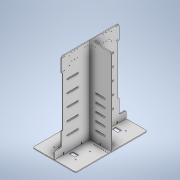
# Autodesk Inventor part: основа
Saved by Autodesk Inventor 2022 (Build 260153000, 153)
## iProperties
Created: 2022-11-18
Part Number: основа
Material: Типовые
Document SubType Name: Modeling
Designer: Ольга
Density: 1 g/cm^3
Appearance: По умолчанию
Author: Ольга
Autodesk Inventor part; units mm, degrees
(part 1 of 2)
sketch "Эскиз1" plane through (0, 0, 0) normal (0, 1, 0) x (-1, 0, 0)
  line L0 (150, 250) -> (-150, 250)
  line L1 (-150, 250) -> (-150, -250)
  line L2 (-150, -250) -> (150, -250)
  line L3 (150, -250) -> (150, 250)
  line L4 (150, 250) -> (-150, -250) construction
  line L5 (-150, 250) -> (150, -250) construction
  line L6 (150, 128.3333) -> (-150, 128.3333) construction
  line L7 (-150, 128.3333) -> (-150, -128.3333) construction
  line L8 (-150, -128.3333) -> (150, -128.3333) construction
  line L9 (150, -128.3333) -> (150, 128.3333) construction
  line L10 (150, 128.3333) -> (-150, -128.3333) construction
  line L11 (-150, 128.3333) -> (150, -128.3333) construction
  line L12 (150, 121.6667) -> (-150, 121.6667) construction
  line L13 (-150, 121.6667) -> (-150, -121.6667) construction
  line L14 (-150, -121.6667) -> (150, -121.6667) construction
  line L15 (150, -121.6667) -> (150, 121.6667) construction
  line L16 (150, 121.6667) -> (-150, -121.6667) construction
  line L17 (-150, 121.6667) -> (150, -121.6667) construction
  line L18 (0, 128.3333) -> (0, 121.6667) construction
  line L19 (0, -121.6667) -> (0, -128.3333) construction
  line L20 (0, 250) -> (0, 125) construction
  line L21 (0, 125) -> (0, 0) construction
  line L22 (0, 0) -> (0, -125) construction
  line L23 (0, -125) -> (0, -250) construction
  circle A0 centre (0, 187.5) radius 2
  circle A1 centre (0, 62.5) radius 2
  circle A2 centre (0, -62.5) radius 2
  circle A3 centre (0, -187.5) radius 2
  line L24 (0, 250) -> (0, 187.5) construction
  line L25 (0, 125) -> (0, 187.5) construction
  line L26 (0, 125) -> (0, 62.5) construction
  line L27 (0, 62.5) -> (0, 0) construction
  line L28 (0, 0) -> (0, -62.5) construction
  line L29 (0, -62.5) -> (0, -125) construction
  line L30 (0, -125) -> (0, -187.5) construction
  line L31 (0, -187.5) -> (0, -250) construction
  line L32 (3, 233.75) -> (-3, 233.75)
  line L33 (-3, 233.75) -> (-3, 203.75)
  line L34 (-3, 203.75) -> (3, 203.75)
  line L35 (3, 203.75) -> (3, 233.75)
  line L36 (3, 233.75) -> (-3, 203.75) construction
  line L37 (-3, 233.75) -> (3, 203.75) construction
  line L38 (3, 171.25) -> (-3, 171.25)
  line L39 (-3, 171.25) -> (-3, 141.25)
  line L40 (-3, 141.25) -> (3, 141.25)
  line L41 (3, 141.25) -> (3, 171.25)
  line L42 (3, 171.25) -> (-3, 141.25) construction
  line L43 (-3, 171.25) -> (3, 141.25) construction
  line L44 (3, 108.75) -> (-3, 108.75)
  line L45 (-3, 108.75) -> (-3, 78.75)
  line L46 (-3, 78.75) -> (3, 78.75)
  line L47 (3, 78.75) -> (3, 108.75)
  line L48 (3, 108.75) -> (-3, 78.75) construction
  line L49 (-3, 108.75) -> (3, 78.75) construction
  line L50 (3, 46.25) -> (-3, 46.25)
  line L51 (-3, 46.25) -> (-3, 16.25)
  line L52 (-3, 16.25) -> (3, 16.25)
  line L53 (3, 16.25) -> (3, 46.25)
  line L54 (3, 46.25) -> (-3, 16.25) construction
  line L55 (-3, 46.25) -> (3, 16.25) construction
  line L56 (3, -16.25) -> (-3, -16.25)
  line L57 (-3, -16.25) -> (-3, -46.25)
  line L58 (-3, -46.25) -> (3, -46.25)
  line L59 (3, -46.25) -> (3, -16.25)
  line L60 (3, -16.25) -> (-3, -46.25) construction
  line L61 (-3, -16.25) -> (3, -46.25) construction
  line L62 (3, -78.75) -> (-3, -78.75)
  line L63 (-3, -78.75) -> (-3, -108.75)
  line L64 (-3, -108.75) -> (3, -108.75)
  line L65 (3, -108.75) -> (3, -78.75)
  line L66 (3, -78.75) -> (-3, -108.75) construction
  line L67 (-3, -78.75) -> (3, -108.75) construction
  line L68 (3, -141.25) -> (-3, -141.25)
  line L69 (-3, -141.25) -> (-3, -171.25)
  line L70 (-3, -171.25) -> (3, -171.25)
  line L71 (3, -171.25) -> (3, -141.25)
  line L72 (3, -141.25) -> (-3, -171.25) construction
  line L73 (-3, -141.25) -> (3, -171.25) construction
  line L74 (3, -203.75) -> (-3, -203.75)
  line L75 (-3, -203.75) -> (-3, -233.75)
  line L76 (-3, -233.75) -> (3, -233.75)
  line L77 (3, -233.75) -> (3, -203.75)
  line L78 (3, -203.75) -> (-3, -233.75) construction
  line L79 (-3, -203.75) -> (3, -233.75) construction
  line L80 (0, 0) -> (-150, 0) construction
  line L81 (-75, 0) -> (0, 0) construction
  line L82 (-75, 0) -> (-150, 0) construction
  line L83 (0, 0) -> (150, 0) construction
  line L84 (75, 0) -> (150, 0) construction
  line L85 (75, 0) -> (0, 0) construction
  line L86 (-97.5, 3) -> (-127.5, 3)
  line L87 (-127.5, 3) -> (-127.5, -3)
  line L88 (-127.5, -3) -> (-97.5, -3)
  line L89 (-97.5, -3) -> (-97.5, 3)
  line L90 (-97.5, 3) -> (-127.5, -3) construction
  line L91 (-127.5, 3) -> (-97.5, -3) construction
  line L92 (-22.5, 3) -> (-52.5, 3)
  line L93 (-52.5, 3) -> (-52.5, -3)
  line L94 (-52.5, -3) -> (-22.5, -3)
  line L95 (-22.5, -3) -> (-22.5, 3)
  line L96 (-22.5, 3) -> (-52.5, -3) construction
  line L97 (-52.5, 3) -> (-22.5, -3) construction
  line L98 (52.5, 3) -> (22.5, 3)
  line L99 (22.5, 3) -> (22.5, -3)
  line L100 (22.5, -3) -> (52.5, -3)
  line L101 (52.5, -3) -> (52.5, 3)
  line L102 (52.5, 3) -> (22.5, -3) construction
  line L103 (22.5, 3) -> (52.5, -3) construction
  line L104 (127.5, 3) -> (97.5, 3)
  line L105 (97.5, 3) -> (97.5, -3)
  line L106 (97.5, -3) -> (127.5, -3)
  line L107 (127.5, -3) -> (127.5, 3)
  line L108 (127.5, 3) -> (97.5, -3) construction
  line L109 (97.5, 3) -> (127.5, -3) construction
  circle A4 centre (-75, 0) radius 2
  circle A5 centre (75, 0) radius 2
  arc A6 (150, 240) -> (140, 250) centre (140, 240) ccw
  arc A7 (140, -250) -> (150, -240) centre (140, -240) ccw
  arc A8 (-150, -240) -> (-140, -250) centre (-140, -240) ccw
  arc A9 (-140, 250) -> (-150, 240) centre (-140, 240) ccw
  line L110 (-150, 20) -> (-8.6161, 20) construction
  circle A10 centre (-140, 20) radius 2.5
  circle A11 centre (-127.1429, 20) radius 2.5
  circle A12 centre (-114.2857, 20) radius 2.5
  circle A13 centre (-101.4286, 20) radius 2.5
  circle A14 centre (-88.5714, 20) radius 2.5
  circle A15 centre (-75.7143, 20) radius 2.5
  circle A16 centre (-62.8571, 20) radius 2.5
  circle A17 centre (-50, 20) radius 2.5
  circle A18 centre (-140, -20) radius 2.5
  circle A19 centre (-127.1429, -20) radius 2.5
  circle A20 centre (-114.2857, -20) radius 2.5
  circle A21 centre (-101.4286, -20) radius 2.5
  circle A22 centre (-88.5714, -20) radius 2.5
  circle A23 centre (-75.7143, -20) radius 2.5
  circle A24 centre (-62.8571, -20) radius 2.5
  circle A25 centre (-50, -20) radius 2.5
  line L111 (0, 125) -> (150, 125) construction
  line L112 (0, -125) -> (150, -125) construction
  circle A26 centre (35, 125) radius 2.5
  circle A27 centre (35, -125) radius 2.5
  point P0 (0, 218.75)
  point P1 (0, 156.25)
  point P2 (0, 93.75)
  point P3 (0, 31.25)
  point P4 (0, -31.25)
  point P5 (0, -93.75)
  point P6 (0, -156.25)
  point P7 (0, -218.75)
  point P8 (0, 156.25)
  point P9 (0, 93.75)
  point P10 (0, 31.25)
  point P11 (0, -31.25)
  point P12 (0, -93.75)
  point P13 (0, -156.25)
  point P14 (0, -218.75)
  point P15 (-112.5, 0)
  point P16 (-37.5, 0)
  point P17 (37.5, 0)
  point P18 (112.5, 0)
  point P19 (-37.5, 0)
  point P20 (37.5, 0)
  point P21 (112.5, 0)
  dimension "d0" = 300
  dimension "d1" = 500
  dimension "d2" = 256.6667
  dimension "d3" = 243.3333
  dimension "d6" = 4
  dimension "d7" = 4
  dimension "d8" = 4
  dimension "d9" = 4
  dimension "d10" = 6
  dimension "d11" = 30
  dimension "d17" = 6
  dimension "d18" = 30
  dimension "d19" = 6
  dimension "d20" = 30
  dimension "d21" = 6
  dimension "d22" = 30
  dimension "d23" = 6
  dimension "d24" = 30
  dimension "d25" = 6
  dimension "d26" = 30
  dimension "d27" = 6
  dimension "d28" = 30
  dimension "d29" = 6
  dimension "d30" = 30
  dimension "d33" = 30
  dimension "d34" = 6
  dimension "d35" = 30
  dimension "d36" = 6
  dimension "d37" = 30
  dimension "d38" = 6
  dimension "d39" = 30
  dimension "d40" = 6
  dimension "d41" = 4
  dimension "d62" = 4
  dimension "d122" = 10
  dimension "d125" = 280
  dimension "d128" = 480
  dimension "d198" = 20
  dimension "d199" = 5
  dimension "d209" = 10
  dimension "d212" = 12.8571
  dimension "d235" = 16.25
  dimension "d236" = 5
  dimension "d237" = 35
  constraints: 226 end point, 58 midpoint, 30 parallel, 28 centre point, 19 horizontal, 17 perpendicular, 15 point on line, 12 collinear, 9 symmetric about line, 8 point on circle, 7 tangent, 5 coincident, 2 vertical, 26 other
  measures "d0" distance of L2.end L1.end
  measures "d1" distance of L1.end L0.end
  measures "d2" distance of L7.end L6.end
  measures "d3" distance of L13.end L12.end
  measures "d6" diameter of A0
  measures "d7" diameter of A1
  measures "d8" diameter of A2
  measures "d9" diameter of A3
  measures "d10" distance of L34.end L33.end
  measures "d11" distance of L33.end L32.end
  measures "d17" distance of L40.end L40.start
  measures "d18" distance of L40.start L39.start
  measures "d19" distance of L46.end L46.start
  measures "d20" distance of L46.start L45.start
  measures "d21" distance of L52.end L52.start
  measures "d22" distance of L52.start L51.start
  measures "d23" distance of L58.end L58.start
  measures "d24" distance of L58.start L57.start
  measures "d25" distance of L64.end L64.start
  measures "d26" distance of L64.start L63.start
  measures "d27" distance of L70.end L70.start
  measures "d28" distance of L70.start L69.start
  measures "d29" distance of L76.end L76.start
  measures "d30" distance of L76.start L75.start
  measures "d33" distance of L88.end L87.end
  measures "d34" distance of L87.end L86.end
  measures "d35" distance of L94.end L94.start
  measures "d36" distance of L94.start L92.end
  measures "d37" distance of L100.end L100.start
  measures "d38" distance of L100.start L98.end
  measures "d39" distance of L106.end L106.start
  measures "d40" distance of L106.start L104.end
  measures "d41" diameter of A4
  measures "d62" diameter of A5
  measures "d122" radius of A6
  measures "d125" distance of A6.centre point (-140, 240)
  measures "d128" distance of A6.centre point (140, -240)
  measures "d198" distance of L110.start L80.end
  measures "d199" diameter of A10
  measures "d209" distance of L110.start A10.centre
  measures "d212" distance of A10.centre A11.centre
  measures "d235" distance from line of L21.end L52
  measures "d236" diameter of A26
  measures "d237" distance of A26.centre L20.end
extrude "Выдавливание1" add sketch "Эскиз1" along normal blind 6 contours A6 L3 A7 L2 A8 L1 A9 L0
ref_plane "РабПлоскость1" through (0, 0, 108.75) normal (1, 0, 0) x (0, 0, -1)
sketch "Эскиз2" plane through (0, 0, 108.75) normal (1, 0, 0) x (0, 0, -1)
  line L0 (294.25, 6) -> (298.25, 6) projected
  line L1 (-80.75, 6) -> (-76.75, 6) construction
  line L2 (348.75, 6) -> (-131.25, 6) construction
  line L3 (44.25, 6) -> (48.25, 6) construction
  line L4 (169.25, 6) -> (173.25, 6) construction
  line L5 (171.25, 6) -> (171.25, 32.7871) construction
  line L6 (46.25, 6) -> (46.25, 27.5686) construction
  line L7 (-80.75, 6) -> (-76.75, 6) construction
  line L8 (-78.75, 6) -> (-78.75, 26.6355) construction
  line L9 (294.25, 6) -> (298.25, 6)
  line L10 (298.25, 6) -> (298.25, 21)
  line L11 (298.25, 21) -> (294.25, 21)
  line L12 (294.25, 21) -> (294.25, 6)
  line L13 (296.25, 21) -> (296.25, 6)
  line L14 (292.83, 12.1) -> (299.67, 12.1)
  line L15 (299.67, 12.1) -> (299.67, 9)
  line L16 (299.67, 9) -> (292.83, 9)
  line L17 (292.83, 9) -> (292.83, 12.1)
  line L18 (292.83, 12.1) -> (299.67, 9) construction
  line L19 (299.67, 12.1) -> (292.83, 9) construction
  line L20 (169.25, 6) -> (173.25, 6)
  line L21 (173.25, 6) -> (173.25, 21)
  line L22 (173.25, 21) -> (169.25, 21)
  line L23 (169.25, 21) -> (169.25, 6)
  line L24 (171.25, 21) -> (171.25, 6)
  line L25 (167.83, 12.1) -> (174.67, 12.1)
  line L26 (174.67, 12.1) -> (174.67, 9)
  line L27 (174.67, 9) -> (167.83, 9)
  line L28 (167.83, 9) -> (167.83, 12.1)
  line L29 (167.83, 12.1) -> (174.67, 9) construction
  line L30 (174.67, 12.1) -> (167.83, 9) construction
  line L31 (44.25, 6) -> (48.25, 6)
  line L32 (48.25, 6) -> (48.25, 21)
  line L33 (48.25, 21) -> (44.25, 21)
  line L34 (44.25, 21) -> (44.25, 6)
  line L35 (46.25, 21) -> (46.25, 6)
  line L36 (42.83, 12.1) -> (49.67, 12.1)
  line L37 (49.67, 12.1) -> (49.67, 9)
  line L38 (49.67, 9) -> (42.83, 9)
  line L39 (42.83, 9) -> (42.83, 12.1)
  line L40 (42.83, 12.1) -> (49.67, 9) construction
  line L41 (49.67, 12.1) -> (42.83, 9) construction
  line L42 (-80.75, 6) -> (-76.75, 6)
  line L43 (-76.75, 6) -> (-76.75, 21)
  line L44 (-76.75, 21) -> (-80.75, 21)
  line L45 (-80.75, 21) -> (-80.75, 6)
  line L46 (-78.75, 21) -> (-78.75, 6)
  line L47 (-82.15, 12.1) -> (-75.35, 12.1)
  line L48 (-75.35, 12.1) -> (-75.35, 9)
  line L49 (-75.35, 9) -> (-82.15, 9)
  line L50 (-82.15, 9) -> (-82.15, 12.1)
  line L51 (-82.15, 12.1) -> (-75.35, 9) construction
  line L52 (-75.35, 12.1) -> (-82.15, 9) construction
  line L53 (-141.25, 6) -> (358.75, 6)
  line L54 (358.75, 6) -> (358.75, 596)
  line L55 (348.75, 606) -> (-131.25, 606)
  line L56 (-141.25, 596) -> (-141.25, 6)
  line L57 (-131.25, 6) -> (348.75, 6) projected
  line L58 (108.75, 606) -> (108.75, 6) construction
  line L59 (-141.25, 6) -> (358.75, 6)
  line L60 (108.75, 606) -> (111.75, 606)
  line L61 (111.75, 606) -> (111.75, 306)
  line L62 (111.75, 306) -> (105.75, 306)
  line L63 (105.75, 306) -> (105.75, 606)
  arc A0 (-131.25, 606) -> (-141.25, 596) centre (-131.25, 596) ccw
  arc A1 (358.75, 596) -> (348.75, 606) centre (348.75, 596) ccw
  point P0 (296.25, 10.55)
  point P1 (171.25, 11.55)
  point P2 (46.25, 11.55)
  point P3 (-78.75, 11.55)
  point P4 (171.25, 10.55)
  point P5 (46.25, 10.55)
  point P6 (-78.75, 10.55)
  point P7 (358.75, 606)
  point P8 (-141.25, 606)
  point P9 (44.25, 12.1)
  point P10 (48.25, 12.1)
  point P11 (48.25, 9)
  point P12 (48.25, 6)
  point P13 (169.25, 9)
  point P14 (169.25, 12.1)
  point P15 (173.25, 12.1)
  point P16 (173.25, 9)
  point P17 (173.25, 6)
  point P18 (294.25, 9)
  point P19 (294.25, 12.1)
  point P20 (298.25, 12.1)
  point P21 (298.25, 9)
  point P22 (-80.75, 9)
  point P23 (-80.75, 12.1)
  point P24 (-76.75, 12.1)
  point P25 (-76.75, 9)
  point P26 (44.25, 6)
  point P27 (44.25, 9)
  point P28 (235.75, 6)
  point P29 (-14.25, 6)
  dimension "d64" = 15
  dimension "d65" = 6.84
  dimension "d66" = 3.1
  dimension "d67" = 3
  dimension "d71" = 15
  dimension "d72" = 6.84
  dimension "d73" = 3.1
  dimension "d74" = 15
  dimension "d75" = 6.84
  dimension "d76" = 3.1
  dimension "d80" = 15
  dimension "d81" = 6.8
  dimension "d82" = 3.1
  dimension "d83" = 600
  dimension "d143" = 3
  dimension "d144" = 300
  dimension "d145" = 6
  dimension "d146" = 300
  dimension "d147" = 3
  dimension "d148" = 3
  dimension "d149" = 3
  dimension "d150" = 10
  dimension "d151" = 10
  constraints: 116 end point, 20 midpoint, 18 parallel, 13 point on line, 11 horizontal, 9 perpendicular, 4 point on circle, 4 tangent, 4 vertical, 2 centre point, 1 collinear, 3 other
  measures "d64" distance of L0.end L10.end
  measures "d65" distance of L15.end L16.end
  measures "d66" distance of L14.end L15.end
  measures "d71" distance of L4.end L21.end
  measures "d72" distance of L26.end L28.start
  measures "d73" distance of L26.start L26.end
  measures "d74" distance of L3.end L32.end
  measures "d75" distance of L37.end L39.start
  measures "d76" distance of L37.start L37.end
  measures "d80" distance of L1.end L43.end
  measures "d81" distance of L48.end L50.start
  measures "d82" distance of L48.start L48.end
  measures "d83" distance of L53.end point (358.75, 606)
  measures "d143" distance of L58.start L60.end
  measures "d144" distance of L60.end L61.end
  measures "d145" distance of L61.end L62.end
  measures "d146" distance of L62.end L63.end
  measures "d147" distance from line of L1.end L49
  measures "d150" radius of A0
  measures "d151" radius of A1
extrude "Выдавливание2" add sketch "Эскиз2" along normal mid plane 6 separate body contours L53 L21 L27 L26 L25 L22 L23 L28 L32 L38 L37 L36 L33 L34 L39 L43 L49 L48 L47 L44 L45 L50 L56 A0 L55 L63 L62 L61 A1 L54 L10 L16 L15 L14 L11 L12 L17
ref_plane "РабПлоскость2" through (22.5, 0, 0) normal (0, 0, 1) x (1, 0, 0)
sketch "Эскиз4" plane through (22.5, 0, 0) normal (0, 0, 1) x (1, 0, 0)
  line L0 (117.5, 6) -> (-162.5, 6) construction
  line L1 (-172.5, 6) -> (127.5, 6)
  line L2 (127.5, 6) -> (127.5, 596)
  line L3 (117.5, 606) -> (-162.5, 606)
  line L4 (-172.5, 596) -> (-172.5, 6)
  line L5 (-19.5, 6) -> (-19.5, 306)
  line L6 (-19.5, 306) -> (-25.5, 306)
  line L7 (-25.5, 306) -> (-25.5, 6)
  arc A0 (-162.5, 606) -> (-172.5, 596) centre (-162.5, 596) ccw
  arc A1 (127.5, 596) -> (117.5, 606) centre (117.5, 596) ccw
  line L8 (-162.5, 6) -> (117.5, 6) projected
  line L9 (-22.5, 606) -> (-22.5, 6) construction
  line L10 (-99.5, 6) -> (-95.5, 6) projected
  line L11 (-99.5, 6) -> (-99.5, 19)
  line L12 (-99.5, 6) -> (-99.5, 0) projected
  line L13 (-99.5, 19) -> (-95.5, 19)
  line L14 (-95.5, 19) -> (-95.5, 6)
  line L15 (-100.9, 12.1) -> (-94.1, 12.1)
  line L16 (-94.1, 12.1) -> (-94.1, 9)
  line L17 (-94.1, 9) -> (-100.9, 9)
  line L18 (-100.9, 9) -> (-100.9, 12.1)
  line L19 (-100.9, 12.1) -> (-94.1, 9) construction
  line L20 (-94.1, 12.1) -> (-100.9, 9) construction
  line L21 (-97.5, 19) -> (-97.5, 6) construction
  line L22 (50.5, 6) -> (50.5, 19)
  line L23 (50.5, 19) -> (54.5, 19)
  line L24 (54.5, 19) -> (54.5, 6)
  line L25 (49.1, 12.1) -> (55.9, 12.1)
  line L26 (55.9, 12.1) -> (55.9, 9)
  line L27 (55.9, 9) -> (49.1, 9)
  line L28 (49.1, 9) -> (49.1, 12.1)
  line L29 (49.1, 12.1) -> (55.9, 9) construction
  line L30 (55.9, 12.1) -> (49.1, 9) construction
  line L31 (52.5, 19) -> (52.5, 6) construction
  line L32 (50.5, 6) -> (54.5, 6) construction
  line L33 (50.5, 6) -> (54.5, 6) construction
  line L34 (50.5, 6) -> (54.5, 6)
  line L35 (-172.5, 0) -> (-172.5, 6) projected
  line L36 (127.5, 0) -> (127.5, 6) projected
  line L37 (-25.5, 606) -> (-19.5, 606) projected
  line L38 (-25.5, 606) -> (-19.5, 606) projected
  line L39 (-19.5, 596) -> (-19.5, 606) projected
  line L40 (-25.5, 606) -> (-19.5, 606)
  point P0 (127.5, 606)
  point P1 (-172.5, 606)
  point P2 (-22.5, 306)
  point P3 (-97.5, 10.55)
  point P4 (-97.5, 10.55)
  point P5 (52.5, 10.55)
  point P6 (52.5, 10.55)
  point P7 (-99.5, 9)
  point P8 (-99.5, 12.1)
  point P9 (-95.5, 12.1)
  point P10 (-95.5, 9)
  point P11 (50.5, 9)
  point P12 (50.5, 12.1)
  point P13 (54.5, 12.1)
  point P14 (54.5, 9)
  dimension "d120" = 10
  dimension "d121" = 10
  dimension "d131" = 13
  dimension "d132" = 6.8
  dimension "d133" = 3.1
  dimension "d134" = 3
  dimension "d135" = 13
  dimension "d136" = 6.8
  dimension "d137" = 3.1
  dimension "d138" = 3
  constraints: 62 end point, 13 midpoint, 7 parallel, 7 point on line, 5 perpendicular, 4 collinear, 4 point on circle, 4 tangent, 3 horizontal, 3 vertical, 2 centre point, 1 other
  measures "d120" radius of A0
  measures "d121" radius of A1
  measures "d131" distance of L10.start L11.end
  measures "d132" distance of L16.end L17.end
  measures "d133" distance of L15.end L16.end
  measures "d134" distance from line of L10.end L17
  measures "d135" distance of L22.start L22.end
  measures "d136" distance of L26.end L30.end
  measures "d137" distance of L26.start L26.end
  measures "d138" distance from line of L24.end L27
extrude "Выдавливание3" add sketch "Эскиз4" along normal mid plane 6 separate body contours L4 A0 L3 A1 L2 L1 L24 L27 L26 L25 L23 L22 L28 L5 L6 L7 L14 L17 L16 L15 L13 L11 L18
sketch "Эскиз5" plane through (-150, 6, 3) normal (0, -1, 0) x (1, 0, 0)
  line L0 (300, 237) -> (300, -243) projected
  line L1 (10, 247) -> (290, 247) projected
  line L2 (0, -243) -> (0, 237) projected
  line L3 (290, -253) -> (10, -253) projected
  circle A0 centre (75, -3) radius 2 projected
  circle A1 centre (225, -3) radius 2 projected
  circle A2 centre (150, -190.5) radius 2 projected
  circle A3 centre (150, -65.5) radius 2 projected
  circle A4 centre (150, 59.5) radius 2 projected
  circle A5 centre (150, 184.5) radius 2 projected
  line L4 (22.5, 0) -> (22.5, -6) projected
  line L5 (52.5, 0) -> (22.5, 0) projected
  line L6 (52.5, -6) -> (52.5, 0) projected
  line L7 (22.5, -6) -> (52.5, -6) projected
  line L8 (97.5, 0) -> (97.5, -6) projected
  line L9 (127.5, 0) -> (97.5, 0) projected
  line L10 (127.5, -6) -> (127.5, 0) projected
  line L11 (97.5, -6) -> (127.5, -6) projected
  line L12 (172.5, 0) -> (172.5, -6) projected
  line L13 (202.5, 0) -> (172.5, 0) projected
  line L14 (202.5, -6) -> (202.5, 0) projected
  line L15 (172.5, -6) -> (202.5, -6) projected
  line L16 (247.5, 0) -> (247.5, -6) projected
  line L17 (277.5, 0) -> (247.5, 0) projected
  line L18 (277.5, -6) -> (277.5, 0) projected
  line L19 (247.5, -6) -> (277.5, -6) projected
  line L20 (153, -236.75) -> (153, -206.75) projected
  line L21 (147, -236.75) -> (153, -236.75) projected
  line L22 (147, -206.75) -> (147, -236.75) projected
  line L23 (153, -206.75) -> (147, -206.75) projected
  line L24 (153, -174.25) -> (153, -144.25) projected
  line L25 (147, -174.25) -> (153, -174.25) projected
  line L26 (147, -144.25) -> (147, -174.25) projected
  line L27 (153, -144.25) -> (147, -144.25) projected
  line L28 (153, -111.75) -> (153, -81.75) projected
  line L29 (147, -111.75) -> (153, -111.75) projected
  line L30 (147, -81.75) -> (147, -111.75) projected
  line L31 (153, -81.75) -> (147, -81.75) projected
  line L32 (153, -49.25) -> (153, -19.25) projected
  line L33 (147, -49.25) -> (153, -49.25) projected
  line L34 (147, -19.25) -> (147, -49.25) projected
  line L35 (153, -19.25) -> (147, -19.25) projected
  line L36 (153, 13.25) -> (153, 43.25) projected
  line L37 (147, 13.25) -> (153, 13.25) projected
  line L38 (147, 43.25) -> (147, 13.25) projected
  line L39 (153, 43.25) -> (147, 43.25) projected
  line L40 (153, 75.75) -> (153, 105.75) projected
  line L41 (147, 75.75) -> (153, 75.75) projected
  line L42 (147, 105.75) -> (147, 75.75) projected
  line L43 (153, 105.75) -> (147, 105.75) projected
  line L44 (153, 138.25) -> (153, 168.25) projected
  line L45 (147, 138.25) -> (153, 138.25) projected
  line L46 (147, 168.25) -> (147, 138.25) projected
  line L47 (153, 168.25) -> (147, 168.25) projected
  line L48 (147, 230.75) -> (147, 200.75) projected
  line L49 (153, 230.75) -> (147, 230.75) projected
  line L50 (153, 200.75) -> (153, 230.75) projected
  line L51 (147, 200.75) -> (153, 200.75) projected
  line L52 (153, -236.75) -> (147, -236.75)
  line L53 (147, -236.75) -> (147, -206.75)
  line L54 (147, -206.75) -> (153, -206.75)
  line L55 (153, -206.75) -> (153, -236.75)
  line L56 (147, -144.25) -> (153, -144.25)
  line L57 (147, -174.25) -> (147, -144.25)
  line L58 (153, -174.25) -> (147, -174.25)
  line L59 (153, -144.25) -> (153, -174.25)
  line L60 (147, -81.75) -> (153, -81.75)
  line L61 (147, -111.75) -> (147, -81.75)
  line L62 (153, -111.75) -> (147, -111.75)
  line L63 (153, -81.75) -> (153, -111.75)
  line L64 (147, -19.25) -> (153, -19.25)
  line L65 (147, -49.25) -> (147, -19.25)
  line L66 (153, -49.25) -> (147, -49.25)
  line L67 (153, -19.25) -> (153, -49.25)
  line L68 (147, 43.25) -> (153, 43.25)
  line L69 (147, 13.25) -> (147, 43.25)
  line L70 (153, 13.25) -> (147, 13.25)
  line L71 (153, 43.25) -> (153, 13.25)
  line L72 (147, 105.75) -> (153, 105.75)
  line L73 (147, 75.75) -> (147, 105.75)
  line L74 (153, 75.75) -> (147, 75.75)
  line L75 (153, 105.75) -> (153, 75.75)
  line L76 (147, 168.25) -> (153, 168.25)
  line L77 (147, 138.25) -> (147, 168.25)
  line L78 (153, 138.25) -> (147, 138.25)
  line L79 (153, 168.25) -> (153, 138.25)
  line L80 (147, 230.75) -> (153, 230.75)
  line L81 (147, 200.75) -> (147, 230.75)
  line L82 (153, 200.75) -> (147, 200.75)
  line L83 (153, 230.75) -> (153, 200.75)
  line L84 (277.5, 0) -> (247.5, 0)
  line L85 (247.5, 0) -> (247.5, -6)
  line L86 (247.5, -6) -> (277.5, -6)
  line L87 (277.5, -6) -> (277.5, 0)
  line L88 (172.5, 0) -> (172.5, -6)
  line L89 (202.5, 0) -> (172.5, 0)
  line L90 (172.5, -6) -> (202.5, -6)
  line L91 (202.5, -6) -> (202.5, 0)
  line L92 (97.5, 0) -> (97.5, -6)
  line L93 (127.5, 0) -> (97.5, 0)
  line L94 (97.5, -6) -> (127.5, -6)
  line L95 (127.5, -6) -> (127.5, 0)
  line L96 (22.5, 0) -> (22.5, -6)
  line L97 (52.5, 0) -> (22.5, 0)
  line L98 (22.5, -6) -> (52.5, -6)
  line L99 (52.5, -6) -> (52.5, 0)
  arc A6 (300, 237) -> (290, 247) centre (290, 237) ccw projected
  arc A7 (10, 247) -> (0, 237) centre (10, 237) ccw projected
  arc A8 (0, -243) -> (10, -253) centre (10, -243) ccw projected
  arc A9 (290, -253) -> (300, -243) centre (290, -243) ccw projected
  point P0 (150, -3)
  dimension "d104" = 62.5
  dimension "d111" = 75
  constraints: 96 end point, 4 parallel, 3 horizontal, 2 coincident, 2 perpendicular, 1 vertical, 80 other
  measures "d104" distance of L22.start L56.start
  measures "d111" distance of L84.end L88.start
extrude "Выдавливание4" add sketch "Эскиз5" along normal up to surface (6 mm away) contours L21 L22 L23 L20 | L25 L26 L27 L24 | L29 L30 L31 L28 | L33 L34 L35 L32 | L37 L38 L39 L36 | L41 L42 L43 L40 | L45 L46 L47 L44 | L49 L50 L51 L48 bodies 2
extrude "Выдавливание5" add sketch "Эскиз5" along normal up to surface (6 mm away) contours L5 L6 L7 L4 | L9 L10 L11 L8 | L13 L14 L15 L12 | L17 L18 L19 L16 bodies 3
sketch "Эскиз6" plane through (22.5, 0, 3) normal (0, 0, 1) x (1, 0, 0)
  line L0 (52.5, 6) -> (52.5, 606) construction
  line L1 (50.5, 6) -> (54.5, 6) construction
  line L2 (50.5, 0) -> (54.5, 0) construction
  line L3 (22.5, 81) -> (82.5, 81) construction
  line L4 (22.5, 76) -> (82.5, 76)
  line L5 (82.5, 86) -> (22.5, 86)
  arc A0 (22.5, 86) -> (22.5, 76) centre (22.5, 81) ccw
  arc A1 (82.5, 76) -> (82.5, 86) centre (82.5, 81) ccw
  line L6 (22.5, 137.25) -> (82.5, 137.25) construction
  line L7 (22.5, 132.25) -> (82.5, 132.25)
  line L8 (82.5, 142.25) -> (22.5, 142.25)
  arc A2 (22.5, 142.25) -> (22.5, 132.25) centre (22.5, 137.25) ccw
  arc A3 (82.5, 132.25) -> (82.5, 142.25) centre (82.5, 137.25) ccw
  line L9 (22.5, 193.5) -> (82.5, 193.5) construction
  line L10 (22.5, 188.5) -> (82.5, 188.5)
  line L11 (82.5, 198.5) -> (22.5, 198.5)
  arc A4 (22.5, 198.5) -> (22.5, 188.5) centre (22.5, 193.5) ccw
  arc A5 (82.5, 188.5) -> (82.5, 198.5) centre (82.5, 193.5) ccw
  line L12 (22.5, 249.75) -> (82.5, 249.75) construction
  line L13 (22.5, 244.75) -> (82.5, 244.75)
  line L14 (82.5, 254.75) -> (22.5, 254.75)
  arc A6 (22.5, 254.75) -> (22.5, 244.75) centre (22.5, 249.75) ccw
  arc A7 (82.5, 244.75) -> (82.5, 254.75) centre (82.5, 249.75) ccw
  line L15 (22.5, 306) -> (82.5, 306) construction
  line L16 (22.5, 301) -> (82.5, 301)
  line L17 (82.5, 311) -> (22.5, 311)
  arc A8 (22.5, 311) -> (22.5, 301) centre (22.5, 306) ccw
  arc A9 (82.5, 301) -> (82.5, 311) centre (82.5, 306) ccw
  line L18 (-162.5, 606) -> (117.5, 606) projected
  point P0 (-22.5, 0)
  point P1 (52.5, 81)
  point P2 (52.5, 137.25)
  point P3 (52.5, 193.5)
  point P4 (52.5, 249.75)
  point P5 (52.5, 306)
  point P6 (52.5, 306)
  dimension "d155" = 70
  dimension "d157" = 60
  dimension "d161" = 56.25
  dimension "d170" = 10
  constraints: 42 end point, 20 point on circle, 10 centre point, 4 midpoint, 4 tangent, 2 point on line, 2 vertical, 1 parallel, 1 perpendicular, 48 other
  measures "d155" distance from line of L0.start L4
  measures "d157" distance of L5.start L5.end
  measures "d161" distance of L4.start L7.start
  measures "d170" distance between parallel lines of L5 L4
extrude "Выдавливание6" cut sketch "Эскиз6" against normal blind 6 bodies 3
sketch "Эскиз7" plane through (3, 0, 108.75) normal (1, 0, 0) x (0, 0, -1)
  line L0 (44.25, 6) -> (48.25, 6) construction
  line L1 (44.25, 0) -> (48.25, 0) construction
  line L2 (-80.75, 6) -> (-76.75, 6) construction
  line L3 (-80.75, 0) -> (-76.75, 0) construction
  line L4 (-76.75, 6) -> (44.25, 6) construction
  line L5 (-16.25, 6) -> (-16.25, 606) construction
  line L6 (-131.25, 606) -> (105.75, 606) construction
  line L7 (-51.25, 451) -> (18.75, 451) construction
  line L8 (-51.25, 446) -> (18.75, 446)
  line L9 (18.75, 456) -> (-51.25, 456)
  arc A0 (-51.25, 456) -> (-51.25, 446) centre (-51.25, 451) ccw
  arc A1 (18.75, 446) -> (18.75, 456) centre (18.75, 451) ccw
  line L10 (-51.25, 361) -> (18.75, 361)
  line L11 (-51.25, 366) -> (18.75, 366) construction
  arc A2 (-51.25, 371) -> (-51.25, 361) centre (-51.25, 366) ccw
  arc A3 (18.75, 361) -> (18.75, 371) centre (18.75, 366) ccw
  line L12 (18.75, 371) -> (-51.25, 371)
  line L13 (-51.25, 276) -> (18.75, 276)
  line L14 (-51.25, 281) -> (18.75, 281) construction
  arc A4 (-51.25, 286) -> (-51.25, 276) centre (-51.25, 281) ccw
  arc A5 (18.75, 276) -> (18.75, 286) centre (18.75, 281) ccw
  line L15 (18.75, 286) -> (-51.25, 286)
  line L16 (-51.25, 191) -> (18.75, 191)
  line L17 (-51.25, 196) -> (18.75, 196) construction
  arc A6 (-51.25, 201) -> (-51.25, 191) centre (-51.25, 196) ccw
  arc A7 (18.75, 191) -> (18.75, 201) centre (18.75, 196) ccw
  line L18 (18.75, 201) -> (-51.25, 201)
  line L19 (-51.25, 106) -> (18.75, 106)
  line L20 (-51.25, 111) -> (18.75, 111) construction
  arc A8 (-51.25, 116) -> (-51.25, 106) centre (-51.25, 111) ccw
  arc A9 (18.75, 106) -> (18.75, 116) centre (18.75, 111) ccw
  line L21 (18.75, 116) -> (-51.25, 116)
  line L22 (198.75, 446) -> (268.75, 446)
  line L23 (198.75, 451) -> (268.75, 451) construction
  arc A10 (198.75, 456) -> (198.75, 446) centre (198.75, 451) ccw
  arc A11 (268.75, 446) -> (268.75, 456) centre (268.75, 451) ccw
  line L24 (268.75, 456) -> (198.75, 456)
  line L25 (198.75, 361) -> (268.75, 361)
  line L26 (198.75, 366) -> (268.75, 366) construction
  arc A12 (198.75, 371) -> (198.75, 361) centre (198.75, 366) ccw
  arc A13 (268.75, 361) -> (268.75, 371) centre (268.75, 366) ccw
  line L27 (268.75, 371) -> (198.75, 371)
  line L28 (198.75, 276) -> (268.75, 276)
  line L29 (198.75, 281) -> (268.75, 281) construction
  arc A14 (198.75, 286) -> (198.75, 276) centre (198.75, 281) ccw
  arc A15 (268.75, 276) -> (268.75, 286) centre (268.75, 281) ccw
  line L30 (268.75, 286) -> (198.75, 286)
  line L31 (198.75, 191) -> (268.75, 191)
  line L32 (198.75, 196) -> (268.75, 196) construction
  arc A16 (198.75, 201) -> (198.75, 191) centre (198.75, 196) ccw
  arc A17 (268.75, 191) -> (268.75, 201) centre (268.75, 196) ccw
  line L33 (268.75, 201) -> (198.75, 201)
  line L34 (198.75, 106) -> (268.75, 106)
  line L35 (198.75, 111) -> (268.75, 111) construction
  arc A18 (198.75, 116) -> (198.75, 106) centre (198.75, 111) ccw
  arc A19 (268.75, 106) -> (268.75, 116) centre (268.75, 111) ccw
  line L36 (268.75, 116) -> (198.75, 116)
  line L37 (233.75, 6) -> (233.75, 658.6053) construction
  line L38 (-76.75, 6) -> (44.25, 6)
  line L39 (348.75, 0) -> (-131.25, 0) projected
  line L40 (173.25, 12.1) -> (173.25, 21) projected
  line L41 (169.25, 6) -> (173.25, 6) projected
  line L42 (294.25, 6) -> (298.25, 6) projected
  line L43 (173.25, 6) -> (294.25, 6)
  point P0 (108.75, 0)
  point P1 (-16.25, 451)
  point P2 (-16.25, 366)
  point P3 (-16.25, 281)
  point P4 (-16.25, 196)
  point P5 (-16.25, 111)
  point P6 (233.75, 451)
  point P7 (233.75, 366)
  point P8 (233.75, 281)
  point P9 (233.75, 196)
  point P10 (233.75, 111)
  point P11 (233.75, 451)
  point P12 (-16.25, 6)
  dimension "d171" = 10
  dimension "d172" = 70
  dimension "d173" = 150
  dimension "d176" = 85
  dimension "d179" = 250
  dimension "d238" = 100
  constraints: 90 end point, 40 point on circle, 20 centre point, 5 midpoint, 4 point on line, 4 tangent, 2 horizontal, 2 parallel, 2 perpendicular, 2 vertical, 108 other
  measures "d171" distance between parallel lines of L8 L9
  measures "d172" distance of L8.start L8.end
  measures "d173" distance between parallel lines of L9 L6
  measures "d176" distance of L8.start L10.start
  measures "d179" distance of L8.start L22.start
  measures "d238" distance between parallel lines of L4 L19
extrude "Выдавливание7" cut sketch "Эскиз7" against normal blind 6 bodies 2
sketch "Эскиз9" plane through (0, 6, 0) normal (0, 1, 0) x (1, 0, 0)
  circle A0 centre (50, -20) radius 2.5 projected
  line L0 (3, -3) -> (3, -240) projected
  line L1 (3, -250) -> (3, -240) projected
  line L2 (-140, -250) -> (140, -250) projected
  arc A1 (140, -250) -> (150, -240) centre (140, -240) ccw projected
  line L3 (150, -240) -> (150, 240) projected
  line L4 (3, -16.25) -> (3, -46.25) construction
  line L5 (3, -22.5) -> (147.0711, -22.5) construction
  line L6 (147.0711, -22.5) -> (147.0711, -247.0711) construction
  line L7 (147.0711, -247.0711) -> (3, -247.0711) construction
  line L8 (3, -247.0711) -> (3, -22.5) construction
  line L9 (137.0711, -32.5) -> (13, -32.5)
  line L10 (13, -32.5) -> (13, -237.0711)
  line L11 (13, -237.0711) -> (137.0711, -237.0711)
  line L12 (137.0711, -237.0711) -> (137.0711, -32.5)
  point P0 (0, 0)
  dimension "d218" = 10
  constraints: 16 end point, 4 parallel, 2 perpendicular, 1 horizontal, 1 point on circle, 1 point on line, 1 tangent, 3 other
  measures "d218" distance between parallel lines of L5 L9
sketch "Эскиз13" plane through (3, 0, 108.75) normal (1, 0, 0) x (0, 0, -1)
  line L0 (198.75, 456) -> (268.75, 456) projected
  arc A0 (268.75, 446) -> (268.75, 456) centre (268.75, 451) ccw projected
  line L1 (268.75, 446) -> (198.75, 446) projected
  arc A1 (198.75, 456) -> (198.75, 446) centre (198.75, 451) ccw projected
  line L2 (198.75, 286) -> (268.75, 286) projected
  arc A2 (268.75, 276) -> (268.75, 286) centre (268.75, 281) ccw projected
  line L3 (268.75, 276) -> (198.75, 276) projected
  arc A3 (198.75, 286) -> (198.75, 276) centre (198.75, 281) ccw projected
  line L4 (-51.25, 456) -> (18.75, 456) projected
  arc A4 (18.75, 446) -> (18.75, 456) centre (18.75, 451) ccw projected
  line L5 (18.75, 446) -> (-51.25, 446) projected
  arc A5 (-51.25, 456) -> (-51.25, 446) centre (-51.25, 451) ccw projected
  line L6 (-51.25, 286) -> (18.75, 286) projected
  arc A6 (18.75, 276) -> (18.75, 286) centre (18.75, 281) ccw projected
  line L7 (18.75, 276) -> (-51.25, 276) projected
  arc A7 (-51.25, 286) -> (-51.25, 276) centre (-51.25, 281) ccw projected
  line L8 (-51.25, 116) -> (18.75, 116) projected
  arc A8 (18.75, 106) -> (18.75, 116) centre (18.75, 111) ccw projected
  line L9 (18.75, 106) -> (-51.25, 106) projected
  arc A9 (-51.25, 116) -> (-51.25, 106) centre (-51.25, 111) ccw projected
  line L10 (-51.25, 201) -> (18.75, 201) projected
  arc A10 (18.75, 191) -> (18.75, 201) centre (18.75, 196) ccw projected
  line L11 (18.75, 191) -> (-51.25, 191) projected
  arc A11 (-51.25, 201) -> (-51.25, 191) centre (-51.25, 196) ccw projected
  line L12 (-51.25, 371) -> (18.75, 371) projected
  arc A12 (18.75, 361) -> (18.75, 371) centre (18.75, 366) ccw projected
  line L13 (18.75, 361) -> (-51.25, 361) projected
  arc A13 (-51.25, 371) -> (-51.25, 361) centre (-51.25, 366) ccw projected
  line L14 (198.75, 201) -> (268.75, 201) projected
  arc A14 (268.75, 191) -> (268.75, 201) centre (268.75, 196) ccw projected
  line L15 (268.75, 191) -> (198.75, 191) projected
  arc A15 (198.75, 201) -> (198.75, 191) centre (198.75, 196) ccw projected
  line L16 (198.75, 371) -> (268.75, 371) projected
  arc A16 (268.75, 361) -> (268.75, 371) centre (268.75, 366) ccw projected
  line L17 (268.75, 361) -> (198.75, 361) projected
  arc A17 (198.75, 371) -> (198.75, 361) centre (198.75, 366) ccw projected
  line L18 (198.75, 116) -> (268.75, 116) projected
  arc A18 (268.75, 106) -> (268.75, 116) centre (268.75, 111) ccw projected
  line L19 (268.75, 106) -> (198.75, 106) projected
  arc A19 (198.75, 116) -> (198.75, 106) centre (198.75, 111) ccw projected
  line L20 (298.25, 6) -> (312.5, 6) projected
  line L21 (312.5, 6) -> (312.5, 0) projected
  line L22 (342.5, 0) -> (312.5, 0) projected
  line L23 (342.5, 6) -> (342.5, 0) projected
  line L24 (342.5, 6) -> (358.75, 6) projected
  line L25 (358.75, 6) -> (358.75, 596) projected
  arc A20 (358.75, 596) -> (348.75, 606) centre (348.75, 596) ccw projected
  line L26 (348.75, 606) -> (111.75, 606) projected
  line L27 (111.75, 606) -> (111.75, 306) projected
  line L28 (111.75, 306) -> (105.75, 306) projected
  line L29 (105.75, 306) -> (105.75, 606) projected
  line L30 (105.75, 606) -> (-131.25, 606) projected
  arc A21 (-131.25, 606) -> (-141.25, 596) centre (-131.25, 596) ccw projected
  line L31 (-141.25, 596) -> (-141.25, 6) projected
  line L32 (-141.25, 6) -> (-125, 6) projected
  line L33 (-125, 6) -> (-125, 0) projected
  line L34 (-95, 0) -> (-125, 0) projected
  line L35 (-95, 6) -> (-95, 0) projected
  line L36 (-95, 6) -> (-80.75, 6) projected
  line L37 (-76.75, 6) -> (-62.5, 6) projected
  line L38 (-62.5, 6) -> (-62.5, 0) projected
  line L39 (-32.5, 0) -> (-62.5, 0) projected
  line L40 (-32.5, 6) -> (-32.5, 0) projected
  line L41 (280, 6) -> (294.25, 6) projected
  line L42 (173.25, 6) -> (187.5, 6) projected
  line L43 (0, 6) -> (0, 0) projected
  line L44 (30, 0) -> (0, 0) projected
  line L45 (30, 6) -> (30, 0) projected
  line L46 (30, 6) -> (44.25, 6) projected
  line L47 (62.5, 6) -> (62.5, 0) projected
  line L48 (92.5, 0) -> (62.5, 0) projected
  line L49 (92.5, 6) -> (92.5, 0) projected
  line L50 (92.5, 6) -> (125, 6) projected
  line L51 (125, 6) -> (125, 0) projected
  line L52 (155, 0) -> (125, 0) projected
  line L53 (155, 6) -> (155, 0) projected
  line L54 (187.5, 6) -> (187.5, 0) projected
  line L55 (217.5, 0) -> (187.5, 0) projected
  line L56 (217.5, 6) -> (217.5, 0) projected
  line L57 (250, 6) -> (250, 0) projected
  line L58 (280, 0) -> (250, 0) projected
  line L59 (280, 6) -> (280, 0) projected
  line L60 (-141.25, 606) -> (-91.25, 606)
  line L61 (-91.25, 596) -> (-91.25, 66)
  line L62 (-101.25, 56) -> (-131.25, 56)
  line L63 (-141.25, 56) -> (-141.25, 606)
  line L64 (-141.25, 596) -> (-141.25, 6) projected
  line L65 (105.75, 606) -> (-131.25, 606) projected
  line L66 (-141.25, 46) -> (-141.25, 19.6406)
  line L67 (-81.25, 606) -> (-14.25, 606)
  arc A22 (-101.25, 56) -> (-91.25, 66) centre (-101.25, 66) ccw
  arc A23 (-81.25, 606) -> (-91.25, 596) centre (-81.25, 596) ccw
  arc A24 (-131.25, 56) -> (-141.25, 46) centre (-131.25, 46) ccw
  line L68 (111.75, 606) -> (105.75, 606) construction
  line L69 (108.75, 606) -> (108.75, 565.581) construction
  arc A25 (358.75, 596) -> (348.75, 606) centre (348.75, 596) ccw
  line L70 (298.25, 21) -> (294.25, 21)
  line L71 (358.75, 606) -> (308.75, 606)
  line L72 (308.75, 596) -> (308.75, 66)
  line L73 (318.75, 56) -> (348.75, 56)
  line L74 (358.75, 56) -> (358.75, 606)
  line L75 (358.75, 46) -> (358.75, 19.6406)
  line L76 (298.75, 606) -> (231.75, 606)
  arc A26 (308.75, 66) -> (318.75, 56) centre (318.75, 66) ccw
  arc A27 (308.75, 596) -> (298.75, 606) centre (298.75, 596) ccw
  arc A28 (358.75, 46) -> (348.75, 56) centre (348.75, 46) ccw
  line L77 (299.67, 9) -> (298.25, 9) projected
  line L78 (298.25, 9) -> (298.25, 6) projected
  line L79 (-80.75, 6) -> (-80.75, 9) projected
  line L80 (-80.75, 9) -> (-82.15, 9) projected
  line L81 (-82.15, 9) -> (-82.15, 12.1) projected
  line L82 (-82.15, 12.1) -> (-80.75, 12.1) projected
  line L83 (-80.75, 12.1) -> (-80.75, 21) projected
  line L84 (-80.75, 21) -> (-76.75, 21) projected
  line L85 (-76.75, 21) -> (-76.75, 12.1) projected
  line L86 (-76.75, 12.1) -> (-75.35, 12.1) projected
  line L87 (-75.35, 12.1) -> (-75.35, 9) projected
  line L88 (-75.35, 9) -> (-76.75, 9) projected
  line L89 (-76.75, 9) -> (-76.75, 6) projected
  line L90 (-32.5, 6) -> (0, 6) projected
  line L91 (44.25, 6) -> (44.25, 9) projected
  line L92 (44.25, 9) -> (42.83, 9) projected
  line L93 (42.83, 9) -> (42.83, 12.1) projected
  line L94 (42.83, 12.1) -> (44.25, 12.1) projected
  line L95 (44.25, 12.1) -> (44.25, 21) projected
  line L96 (44.25, 21) -> (48.25, 21) projected
  line L97 (48.25, 21) -> (48.25, 12.1) projected
  line L98 (48.25, 12.1) -> (49.67, 12.1) projected
  line L99 (49.67, 12.1) -> (49.67, 9) projected
  line L100 (49.67, 9) -> (48.25, 9) projected
  line L101 (48.25, 9) -> (48.25, 6) projected
  line L102 (48.25, 6) -> (62.5, 6) projected
  line L103 (155, 6) -> (169.25, 6) projected
  line L104 (169.25, 6) -> (169.25, 9) projected
  line L105 (169.25, 9) -> (167.83, 9) projected
  line L106 (167.83, 9) -> (167.83, 12.1) projected
  line L107 (167.83, 12.1) -> (169.25, 12.1) projected
  line L108 (169.25, 12.1) -> (169.25, 21) projected
  line L109 (169.25, 21) -> (173.25, 21) projected
  line L110 (173.25, 21) -> (173.25, 12.1) projected
  line L111 (173.25, 12.1) -> (174.67, 12.1) projected
  line L112 (174.67, 12.1) -> (174.67, 9) projected
  line L113 (174.67, 9) -> (173.25, 9) projected
  line L114 (173.25, 9) -> (173.25, 6) projected
  line L115 (217.5, 6) -> (250, 6) projected
  line L116 (294.25, 6) -> (294.25, 9) projected
  line L117 (294.25, 9) -> (292.83, 9) projected
  line L118 (292.83, 9) -> (292.83, 12.1) projected
  line L119 (292.83, 12.1) -> (294.25, 12.1) projected
  line L120 (294.25, 12.1) -> (294.25, 21) projected
  line L121 (294.25, 21) -> (298.25, 21) projected
  line L122 (298.25, 21) -> (298.25, 12.1) projected
  line L123 (298.25, 12.1) -> (299.67, 12.1) projected
  line L124 (299.67, 12.1) -> (299.67, 9) projected
  point P0 (108.75, 0)
  point P1 (-91.25, 56)
  point P2 (308.75, 56)
  point P3 (-141.25, 46)
  dimension "d223" = 50
  dimension "d224" = 550
  dimension "d225" = 10
  dimension "d226" = 10
  constraints: 28 end point, 16 symmetric about line, 14 point on circle, 14 point on line, 7 centre point, 6 tangent, 2 collinear, 2 parallel, 1 equal radius, 1 horizontal, 1 midpoint, 1 perpendicular, 1 vertical, 4 other
  measures "d223" distance of point (-91.25, 56) L63.start
  measures "d224" distance of L60.end point (-91.25, 56)
  measures "d225" radius of A22
  measures "d226" radius of A23
extrude "Выдавливание11" cut sketch "Эскиз13" against normal up to surface (6 mm away) contours A28 L73 A26 L72 A27 L26 A20 L25 | A23 L61 A22 L62 A24 L31 A21 L30 bodies 2
sketch "Эскиз15" plane through (22.5, 0, 3) normal (0, 0, 1) x (1, 0, 0)
  line L0 (-19.5, 606) -> (-19.5, 306) projected
  line L1 (-19.5, 606) -> (126.0275, 368.404)
  line L2 (127.5, 6) -> (127.5, 596) projected
  line L3 (127.5, 363.1809) -> (127.5, 351.8775)
  line L4 (-19.5, 606) -> (-27.8702, 606)
  line L5 (117.5, 606) -> (-162.5, 606) projected
  arc A0 (127.5, 363.1809) -> (126.0275, 368.404) centre (117.5, 363.1809) ccw
  line L6 (-19.5, 606) -> (127.5, 606)
  line L7 (127.5, 606) -> (127.5, 363.1809)
  line L8 (-25.5, 606) -> (-19.5, 606) construction
  line L9 (-22.5, 606) -> (-22.5, 569.2816) construction
  line L10 (-25.5, 606) -> (-171.0275, 368.404)
  line L11 (-172.5, 6) -> (-172.5, 596)
  line L12 (-162.5, 606) -> (117.5, 606)
  line L13 (-25.5, 606) -> (-172.5, 606)
  line L14 (-172.5, 606) -> (-172.5, 363.1809)
  arc A1 (-171.0275, 368.404) -> (-172.5, 363.1809) centre (-162.5, 363.1809) ccw
  point P0 (-22.5, 0)
  point P1 (127.5, 366)
  dimension "d231" = 230
  dimension "d232" = 10
  constraints: 22 end point, 9 symmetric about line, 6 point on line, 4 point on circle, 2 centre point, 2 tangent, 1 horizontal, 1 midpoint, 1 vertical, 1 other
  measures "d231" distance of L2.end point (127.5, 366)
  measures "d232" radius of A0
extrude "Выдавливание13" cut sketch "Эскиз15" against normal up to surface (6 mm away) contours L10 A1 L11 L14 L13 L5 L4 bodies 3
sketch "Эскиз16" plane through (3, 0, 108.75) normal (1, 0, 0) x (0, 0, -1)
  line L0 (111.75, 606) -> (105.75, 606) projected
  line L1 (105.75, 596) -> (105.75, 606) projected
  line L2 (111.75, 596) -> (105.75, 596) projected
  line L3 (111.75, 606) -> (111.75, 596) projected
  line L4 (-81.25, 606) -> (105.75, 606) construction
  line L5 (105.75, 606) -> (105.75, 583.5) construction
  line L6 (105.75, 6) -> (105.75, 596) construction
  line L7 (105.75, 583.5) -> (91.25, 583.5) construction
  line L8 (91.25, 583.5) -> (71.25, 583.5) construction
  circle A0 centre (71.25, 583.5) radius 2
  circle A1 centre (91.25, 583.5) radius 2
  line L9 (108.75, 606) -> (108.75, 583.5) construction
  circle A2 centre (146.25, 583.5) radius 2
  circle A3 centre (126.25, 583.5) radius 2
  point P0 (108.75, 0)
  dimension "d239" = 22.5
  dimension "d240" = 14.5
  dimension "d241" = 20
  dimension "d242" = 4
  dimension "d243" = 4
  constraints: 8 end point, 4 centre point, 2 coincident, 2 point on line, 2 symmetric about line, 1 midpoint, 1 perpendicular, 1 vertical, 2 other
  measures "d239" distance of L0.end L5.end
  measures "d240" distance of L5.end L7.end
  measures "d241" distance of L7.end L8.end
  measures "d242" diameter of A0
  measures "d243" diameter of A1
sketch "Эскиз17" plane through (22.5, 0, 3) normal (0, 0, 1) x (1, 0, 0)
  line L0 (-19.5, 581.5) -> (-19.5, 585.5) projected
  line L1 (-19.5, 583.5) -> (-5, 583.5) construction
  line L2 (-5, 583.5) -> (15, 583.5) construction
  circle A0 centre (-5, 583.5) radius 2
  circle A1 centre (15, 583.5) radius 2
  point P0 (-22.5, 0)
  dimension "d244" = 14.5
  dimension "d245" = 20
  dimension "d246" = 4
  dimension "d247" = 4
  constraints: 4 end point, 2 centre point, 2 coincident, 2 horizontal, 1 midpoint
  measures "d244" distance of L1.start L1.end
  measures "d245" distance of L1.end L2.end
  measures "d246" diameter of A0
  measures "d247" diameter of A1
extrude "Выдавливание14" cut sketch "Эскиз16" against normal up to surface (6 mm away) contours A0 | A1 | A2 | A3 bodies 2
extrude "Выдавливание15" cut sketch "Эскиз17" against normal up to surface (6 mm away) bodies 3
ref_plane "РабПлоскость3" through (22.5, 0, 0) normal (0, 0, -1) x (-1, 0, 0)
sketch "Эскиз18" plane through (3, 0, 108.75) normal (1, 0, 0) x (0, 0, -1)
  line L0 (-91.25, 66) -> (-91.25, 596) projected
  line L1 (-89.25, 506) -> (-85.75, 506)
  line L2 (-83.75, 504) -> (-83.75, 158)
  line L3 (-85.75, 156) -> (-89.25, 156)
  line L4 (-91.25, 156) -> (-91.25, 506)
  line L5 (105.75, 606) -> (-81.25, 606) projected
  arc A0 (-83.75, 504) -> (-85.75, 506) centre (-85.75, 504) ccw
  line L6 (-91.25, 508) -> (-91.25, 531.208)
  arc A1 (-91.25, 508) -> (-89.25, 506) centre (-89.25, 508) ccw
  arc A2 (-85.75, 156) -> (-83.75, 158) centre (-85.75, 158) ccw
  line L7 (-91.25, 154) -> (-91.25, 127.391)
  arc A3 (-89.25, 156) -> (-91.25, 154) centre (-89.25, 154) ccw
  line L8 (108.75, 727.2) -> (108.75, -121.2) projected
  line L9 (308.75, 66) -> (308.75, 596)
  line L10 (306.75, 506) -> (303.25, 506)
  line L11 (301.25, 504) -> (301.25, 158)
  line L12 (303.25, 156) -> (306.75, 156)
  arc A4 (303.25, 506) -> (301.25, 504) centre (303.25, 504) ccw
  arc A5 (306.75, 506) -> (308.75, 508) centre (306.75, 508) ccw
  arc A6 (301.25, 158) -> (303.25, 156) centre (303.25, 158) ccw
  arc A7 (308.75, 154) -> (306.75, 156) centre (306.75, 154) ccw
  point P0 (108.75, 0)
  point P1 (-83.75, 156)
  point P2 (-83.75, 506)
  point P3 (308.75, 508)
  point P4 (-91.25, 508)
  point P5 (-91.25, 154)
  dimension "d266" = 7.5
  dimension "d267" = 100
  dimension "d268" = 350
  dimension "d269" = 2
  dimension "d270" = 2
  dimension "d271" = 2
  constraints: 20 end point, 16 point on circle, 14 symmetric about line, 11 point on line, 8 centre point, 8 tangent, 2 parallel, 1 equal radius, 1 horizontal, 1 perpendicular, 4 other
  measures "d266" distance between parallel lines of L0 L2
  measures "d267" distance between parallel lines of L1 L5
  measures "d268" distance of point (-83.75, 506) point (-83.75, 156)
  measures "d269" radius of A0
  measures "d270" radius of A1
  measures "d271" radius of A3
extrude "Выдавливание16" cut sketch "Эскиз18" against normal up to surface (6 mm away) bodies 2
sketch "Эскиз19" plane through (22.5, 0, 3) normal (0, 0, 1) x (1, 0, 0)
  point P0 (-22.5, 0)
sketch "Эскиз20" plane through (0, 6, 0) normal (0, 1, 0) x (1, 0, 0)
  line L0 (0, 0) -> (150, 0) construction
  line L1 (150, -240) -> (150, 240) construction
  line L2 (-140, -250) -> (140, -250) construction
  line L3 (0, -250) -> (0, 0) construction
  line L4 (75, -125) -> (75, -175) construction
  line L5 (75, -125) -> (75, -75) construction
  circle A0 centre (75, -175) radius 3
  circle A1 centre (75, -75) radius 3
  line L6 (-75, -125) -> (-75, -175) construction
  line L7 (-75, -125) -> (-75, -75) construction
  circle A2 centre (-75, -175) radius 3
  circle A3 centre (-75, -75) radius 3
  line L8 (75, 125) -> (75, 75) construction
  line L9 (75, 125) -> (75, 175) construction
  circle A4 centre (75, 75) radius 3
  circle A5 centre (75, 175) radius 3
  line L10 (-75, 125) -> (-75, 75) construction
  line L11 (-75, 125) -> (-75, 175) construction
  circle A6 centre (-75, 75) radius 3
  circle A7 centre (-75, 175) radius 3
  dimension "d274" = 50
  dimension "d275" = 50
  dimension "d276" = 6
  dimension "d277" = 6
  dimension "d280" = 150
  dimension "d283" = 250
  constraints: 20 end point, 8 centre point, 8 coincident, 3 vertical, 2 midpoint, 1 horizontal, 1 perpendicular, 27 other
  measures "d274" distance of L4.start L4.end
  measures "d275" distance of L4.start L5.end
  measures "d276" diameter of A0
  measures "d277" diameter of A1
  measures "d280" distance of L4.start L6.start
  measures "d283" distance of L4.start L8.start
extrude "Выдавливание17" cut sketch "Эскиз20" against normal blind 6 bodies 1